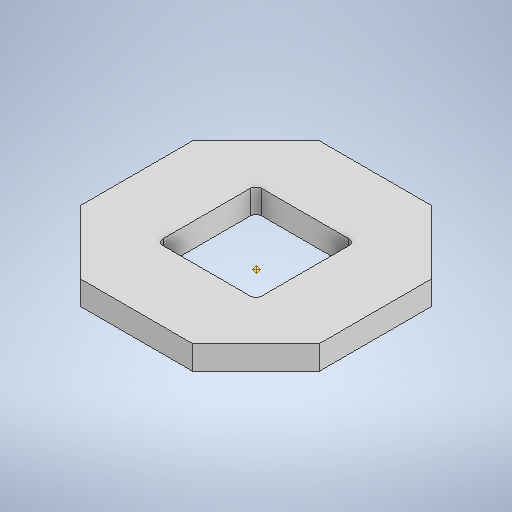
# Autodesk Inventor part: chamber_top
Saved by Autodesk Inventor 2025.4 (Build 294407000, 407)
## iProperties
Created: 2026-05-14
Part Number: chamber_top
Material: Generic
Document SubType Name: Sheet Metal
Designer: zboichykb
Density: 1 g/cm^3
Appearance: Default
Sheet Metal Rule: Default
Author: zboichykb
Autodesk Inventor part; units mm, degrees
ref_plane "YZ Plane" through (0, 0, 0) normal (1, 0, 0) x (0, 1, 0)
ref_plane "XZ Plane" through (0, 0, 0) normal (0, 1, 0) x (-1, 0, 0)
ref_plane "XY Plane" through (0, 0, 0) normal (0, 0, 1) x (1, 0, 0)
sketch "Sketch1" plane through (0, 0, 0) normal (0, 1, 0) x (-1, 0, 0)
  line L0 (0, 0) -> (254, 0)
  line L1 (254, 0) -> (254, -119.38)
  line L2 (254, -119.38) -> (0, -119.38)
  line L3 (0, -119.38) -> (0, 0)
  line L4 (186.69, 67.31) -> (67.31, 67.31)
  line L5 (67.31, 67.31) -> (67.31, -186.69)
  line L6 (67.31, -186.69) -> (186.69, -186.69)
  line L7 (186.69, -186.69) -> (186.69, 67.31)
  line L8 (186.69, 67.31) -> (254, 0)
  line L9 (67.31, 67.31) -> (0, 0)
  line L10 (186.69, -186.69) -> (254, -119.38)
  line L11 (0, -119.38) -> (67.31, -186.69)
  line L12 (62.2907, -7.1202) -> (161.0967, -7.1202)
  line L13 (164.2717, -10.2952) -> (164.2717, -109.1012)
  line L14 (161.0967, -112.2762) -> (62.2907, -112.2762)
  line L15 (59.1157, -109.1012) -> (59.1157, -10.2952)
  arc A0 (62.2907, -7.1202) -> (59.1157, -10.2952) centre (62.2907, -10.2952) ccw
  arc A1 (164.2717, -10.2952) -> (161.0967, -7.1202) centre (161.0967, -10.2952) ccw
  arc A2 (161.0967, -112.2762) -> (164.2717, -109.1012) centre (161.0967, -109.1012) ccw
  arc A3 (59.1157, -109.1012) -> (62.2907, -112.2762) centre (62.2907, -109.1012) ccw
  line L16 (254, -119.38) -> (127, -119.38)
  line L17 (126.9917, -59.69) -> (127, -119.38)
  point P0 (164.2717, -112.2762)
  point P1 (164.2717, -7.1202)
  point P2 (59.1157, -112.2762)
  point P3 (127, -59.69)
  point P4 (127, -59.69)
  dimension "d0" = 254
  dimension "d1" = 119.38
  dimension "d2" = 119.38
  dimension "d3" = 254
  dimension "d8" = 95.1907
  dimension "d14" = 105.156
  dimension "d15" = 105.156
  dimension "d22" = 3.175
  dimension "d50" = 127
  dimension "d51" = 59.69
  constraints: 36 end point, 8 point on circle, 8 tangent, 7 coincident, 7 parallel, 6 point on line, 4 centre point, 4 horizontal, 3 equal radius, 3 perpendicular
  measures "d0" distance of L1.end L2.end
  measures "d1" distance of L0.end L1.end
  measures "d2" distance of L6.end L5.end
  measures "d3" distance of L5.end L4.end
  measures "d8" distance of L0.end L4.start
  measures "d14" distance of point (164.272, -112.276) point (59.116, -112.276)
  measures "d15" distance of point (164.272, -7.12) point (164.272, -112.276)
  measures "d22" radius of A0
  measures "d50" distance of L16.start L16.end
  measures "d51" distance of L17.start L17.end
extrude "Extrusion1" add sketch "Sketch1" along normal blind 25.4
sketch "Sketch3" plane through (0, 0, 0) normal (0, -1, 0) x (1, 0, 0)
  line L0 (-80.7772, -112.268) -> (-173.2332, -112.268)
  line L1 (-179.5832, -105.918) -> (-179.5832, -13.462)
  line L2 (-173.2332, -7.112) -> (-80.7772, -7.112)
  line L3 (-74.4272, -13.462) -> (-74.4272, -105.918)
  arc A0 (-80.7772, -112.268) -> (-74.4272, -105.918) centre (-80.7772, -105.918) ccw
  arc A1 (-179.5832, -105.918) -> (-173.2332, -112.268) centre (-173.2332, -105.918) ccw
  arc A2 (-173.2332, -7.112) -> (-179.5832, -13.462) centre (-173.2332, -13.462) ccw
  arc A3 (-74.4272, -13.462) -> (-80.7772, -7.112) centre (-80.7772, -13.462) ccw
  line L4 (-124.213, 67.31) -> (-124.213, -7.112)
  line L5 (-254.0007, -58.0211) -> (-179.5787, -58.0211)
  line L6 (-186.69, 67.31) -> (-67.31, 67.31) projected
  point P0 (0, 0)
  point P1 (-179.5832, -7.112)
  point P2 (-179.5832, -112.268)
  point P3 (-74.4272, -7.112)
  point P4 (-179.5832, -58.0211)
  dimension "d23" = 105.156
  dimension "d24" = 105.156
  dimension "d42" = 6.35
  dimension "d45" = 74.422
  dimension "d46" = 74.422
  constraints: 12 end point, 10 point on line, 8 point on circle, 8 tangent, 7 coincident, 4 centre point, 3 equal radius, 2 horizontal, 2 parallel, 2 perpendicular, 1 vertical
  measures "d23" distance of point (-179.583, -7.112) point (-74.427, -7.112)
  measures "d24" distance of point (-179.583, -112.268) point (-179.583, -7.112)
  measures "d42" radius of A0
  measures "d45" distance of L4.start L4.end
  measures "d46" distance of L5.start L5.end
extrude "Extrusion2" cut sketch "Sketch3" against normal blind 25.4
equation "\"d0\" = rectangle_L"
equation "\"d1\" = rectangle_01_w"
equation "\"d2\" = rectangle_01_w"
equation "\"d3\" = rectangle_L"
equation "\"d8\" = d9"
equation "\"d14\" = window_L"
equation "\"d15\" = window_L"
equation "\"rectangle_L\" = 254"
equation "\"rectangle_01_w\" = 119.38"
equation "\"d9\" = 95.19071"
equation "\"window_L\" = 105.156"
equation "\"test\" = 74.422"
equation "\"d47\" = 74.422"
equation "\"d48\" = 254"
equation "\"d49\" = 105.156"
equation "\"dot_pos\" = 127"
equation "\"dot_pos_2\" = 59.69"
body "Solid1"
